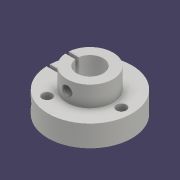
# Autodesk Inventor part: AA056
Saved by Autodesk Inventor 2017 SP1 (Build 210196100, 196)
## iProperties
Created: 2018-06-25
Part Number: AA056
Material: Aluminum 6061
Document SubType Name: Modeling
Designer: Zach
Density: 2.7 g/cm^3
Appearance: Aluminum - Flat
Author: Zach
Autodesk Inventor part; units mm, degrees
ref_plane "YZ Plane" through (0, 0, 0) normal (1, 0, 0) x (0, 1, 0)
ref_plane "XZ Plane" through (0, 0, 0) normal (0, 1, 0) x (-1, 0, 0)
ref_plane "XY Plane" through (0, 0, 0) normal (0, 0, 1) x (1, 0, 0)
sketch "Sketch1" plane through (0, 0, 0) normal (0, 0, 1) x (1, 0, 0)
  circle A0 centre (0, 0) radius 12.7
  circle A1 centre (0, 0) radius 4
  circle A2 centre (9.525, 0) radius 1.5
  circle A3 centre (-4.7625, 8.2489) radius 1.5
  circle A4 centre (-4.7625, -8.2489) radius 1.5
  dimension "d0" = 25.4
  dimension "d1" = 8
  dimension "d2" = 3
  dimension "d6" = 360
  dimension "d25" = 9.525
  constraints: 5 centre point, 3 coincident, 1 horizontal alignment, 7 other
  measures "d0" diameter of A0
  measures "d1" diameter of A1
  measures "d2" diameter of A2
  measures "d25" distance of point (0, 0) A2.centre
extrude "Extrusion1" add sketch "Sketch1" along normal blind 12.7
sketch "Sketch2" plane through (0, 0, 12.7) normal (0, 0, 1) x (1, 0, 0)
  line L0 (-12.7, 0.5) -> (-3.9686, 0.5)
  line L1 (-3.9686, 0.5) -> (-3.9686, -0.5)
  line L2 (-3.9686, -0.5) -> (-12.7, -0.5)
  line L3 (-12.7, -0.5) -> (-12.7, 0.5)
  circle A0 centre (0, 0) radius 12.7 construction
  circle A1 centre (0, 0) radius 4 construction
  point P0 (-3.9686, 0)
  point P1 (-12.7, 0)
  dimension "d10" = 1
  constraints: 8 end point, 2 horizontal alignment, 2 midpoint, 2 parallel, 1 horizontal, 1 perpendicular, 3 other
  measures "d10" distance of L2.end L0.start
extrude "Extrusion2" cut sketch "Sketch2" against normal through all
sketch "Sketch3" plane through (-12.6902, 0.5, 12.7) normal (0, -1, 0) x (1, 0, 0)
  circle A0 centre (3, -3) radius 2
  circle A1 centre (3, -9.45) radius 2
  line L0 (25.3902, 0) -> (0, 0) projected
  line L1 (0, -12.7) -> (25.3902, -12.7) projected
  point P0 (12.6902, -12.7)
  point P1 (12.6902, -12.7)
  point P2 (12.6902, -12.7)
  point P3 (12.6902, -12.7)
  point P4 (12.6902, -12.7)
  dimension "d13" = 4
  dimension "d14" = 4
  dimension "d15" = 3
  dimension "d16" = 3
  dimension "d17" = 3.25
  constraints: 2 centre point, 2 coincident, 1 vertical alignment
  measures "d13" diameter of A0
  measures "d14" diameter of A1
  measures "d15" horizontal distance of L0.end A0.centre
  measures "d16" distance from line of L0 A0.centre
  measures "d17" distance from line of L1 A1.centre
extrude "Extrusion3" cut sketch "Sketch3" along normal through all both and the other way through all
sketch "Sketch4" plane through (0, 0, 12.7) normal (0, 0, 1) x (1, 0, 0)
  circle A0 centre (0, 0) radius 7
  arc A1 (-12.6902, -0.5) -> (-12.6902, 0.5) centre (0, 0) ccw projected
  circle A2 centre (0, 0) radius 12.7
  dimension "d24" = 14
  constraints: 2 coincident, 1 centre point, 3 other
  measures "d24" diameter of A0
extrude "Extrusion4" cut sketch "Sketch4" against normal blind 6.2
sketch "Sketch5" plane through (0, 0, 0) normal (0, 1, 0) x (-1, 0, 0)
  circle A0 centre (0, 9.6) radius 1.5
  circle A1 centre (0, 3.25) radius 1.5
  line L0 (-12.7, 0) -> (-12.7, 6.5) projected
  line L1 (-7, 12.7) -> (-7, 6.5) projected
  point P0 (0, 0)
  point P1 (-12.7, 3.25)
  point P2 (-7, 9.6)
  dimension "d28" = 3
  dimension "d29" = 3
  constraints: 2 centre point, 2 horizontal alignment, 2 midpoint, 2 vertical alignment
  measures "d28" diameter of A0
  measures "d29" diameter of A1
extrude "Extrusion5" cut sketch "Sketch5" against normal through all contours A0
thread "Thread2" size "M4x0.7" class "6H" standard "ANSI Metric M Profile" full length
thread "Thread3" size "M3x0.5" class "6H" standard "ANSI Metric M Profile" full length
body "Solid1"
